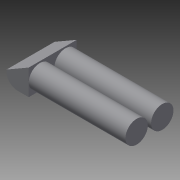
# Autodesk Inventor part: DMJ_Legs
Saved by Autodesk Inventor 2015 SP1 (Build 190203100, 203)
## iProperties
Created: 2016-02-03
Part Number: DMJ_Legs
Material: Generic
Document SubType Name: Modeling
Designer: guillemd
Density: 0.665801 g/cm^3
Appearance: Default
Mass: 31751.5 g
Surface Area: 11536.8 cm^2
Volume: 47689.2 cm^3
Author: guillemd
Autodesk Inventor part; units mm, degrees
ref_plane "YZ Plane" through (0, 0, 0) normal (1, 0, 0) x (0, 1, 0)
ref_plane "XZ Plane" through (0, 0, 0) normal (0, 1, 0) x (-1, 0, 0)
ref_plane "XY Plane" through (0, 0, 0) normal (0, 0, 1) x (1, 0, 0)
sketch "Sketch1" plane through (0, 0, 0) normal (0, 0, 1) x (1, 0, 0)
  line L0 (0, 203.2) -> (0, 0)
  line L1 (0, 0) -> (-88.9, 0)
  line L2 (-175.9764, 101.6) -> (-175.9764, 87.0764)
  arc A0 (-175.9764, 87.0764) -> (-88.9, 0) centre (-88.9, 87.0764) ccw
  line L3 (-175.9764, 101.6) -> (0, 203.2)
  line L4 (0, -62.2809) -> (0, 247.4468) projected
  dimension "d1" = 203.2
  dimension "d2" = 60
  dimension "d3" = 203.2
  dimension "d4" = 88.9
  constraints: 8 end point, 2 perpendicular, 2 point on circle, 2 tangent, 1 centre point, 1 coincident, 1 horizontal, 1 point on line
  measures "d1" distance of L0.start L2.start
  measures "d2" angle of L0 L3
  measures "d3" distance of L0.start L0.end
  measures "d4" horizontal distance of point (0, 0) A0.centre
extrude "Extrusion1" add sketch "Sketch1" along normal mid plane 381
sketch "Sketch2" plane through (0, 0, 190.5) normal (1, 0, 0) x (0, 0, -1)
  line L0 (0, 101.6) -> (381, 101.6) projected
  circle A0 centre (88.9, 101.6) radius 88.9
  circle A1 centre (292.1, 101.6) radius 88.9
  point P0 (190.5, 0)
  dimension "d7" = 177.8
  dimension "d8" = 177.8
  constraints: 2 horizontal alignment, 2 point on line, 4 other
extrude "Extrusion2" add sketch "Sketch2" along normal blind 767.08
body "Solid1"
